Autodesk Fusion 360 part; units mm, degrees
(part 2 of 2)
sketch "Sketch5" plane through (0, 0, 12.2) normal (0, 0, 1) x (-1, 0, 0)
  circle A0 centre (8.13, -15.47) radius 0.762
  circle A1 centre (10.67, -18.01) radius 0.762
  circle A2 centre (8.13, -20.55) radius 0.762
  circle A3 centre (10.67, -23.09) radius 0.762
  circle A4 centre (8.13, -28.17) radius 0.762
  circle A5 centre (10.67, -25.63) radius 0.762
  circle A6 centre (10.67, -30.71) radius 0.762
  circle A7 centre (8.13, -33.25) radius 0.762
  circle A8 centre (10.67, -35.79) radius 0.762
  circle A9 centre (8.13, -38.33) radius 0.762
  circle A10 centre (13.21, -38.33) radius 0.762
  circle A11 centre (13.21, -33.25) radius 0.762
  circle A12 centre (13.21, -28.17) radius 0.762
  circle A13 centre (13.21, -23.09) radius 0.762
  circle A14 centre (13.21, -18.01) radius 0.762
  circle A15 centre (13.21, -12.93) radius 0.762
  circle A16 centre (8.13, -12.93) radius 0.762
  circle A17 centre (10.67, -10.39) radius 0.762
  circle A18 centre (13.21, -7.85) radius 0.762
  circle A19 centre (8.13, -7.85) radius 0.762
  circle A20 centre (5.59, -10.39) radius 0.762
  circle A21 centre (5.59, -15.47) radius 0.762
  circle A22 centre (5.59, -20.55) radius 0.762
  circle A23 centre (5.59, -25.63) radius 0.762
  circle A24 centre (5.59, -30.71) radius 0.762
  circle A25 centre (5.59, -35.79) radius 0.762
  circle A26 centre (3.05, -38.33) radius 0.762
  circle A27 centre (3.05, -33.25) radius 0.762
  circle A28 centre (3.05, -28.17) radius 0.762
  circle A29 centre (3.05, -23.09) radius 0.762
  circle A30 centre (3.05, -18.01) radius 0.762
  circle A31 centre (3.05, -12.93) radius 0.762
  circle A32 centre (3.05, -7.85) radius 0.762
  circle A33 centre (3.05, -5.31) radius 0.762
  circle A34 centre (5.59, -2.77) radius 0.762
  circle A35 centre (8.13, -5.31) radius 0.762
  circle A36 centre (13.21, -5.31) radius 0.762
  circle A37 centre (13.21, -2.77) radius 0.762
  circle A38 centre (13.21, 4.85) radius 0.762
  circle A39 centre (13.21, 7.39) radius 0.762
  circle A40 centre (10.67, 7.39) radius 0.762
  circle A41 centre (10.67, -0.23) radius 0.762
  circle A42 centre (8.13, 2.31) radius 0.762
  circle A43 centre (8.13, 7.39) radius 0.762
  circle A44 centre (5.59, 4.85) radius 0.762
  circle A45 centre (5.59, -0.23) radius 0.762
  circle A46 centre (3.05, -0.23) radius 0.762
  circle A47 centre (3.05, 7.39) radius 0.762
  circle A48 centre (5.59, 9.93) radius 0.762
  circle A49 centre (10.67, 9.93) radius 0.762
  circle A50 centre (13.21, 12.47) radius 0.762
  circle A51 centre (8.13, 12.47) radius 0.762
  circle A52 centre (8.13, 15.01) radius 0.762
  circle A53 centre (13.21, 15.01) radius 0.762
  circle A54 centre (13.21, 17.55) radius 0.762
  circle A55 centre (5.59, 20.09) radius 0.762
  circle A56 centre (8.13, 20.09) radius 0.762
  circle A57 centre (8.13, 22.63) radius 0.762
  circle A58 centre (3.05, 22.63) radius 0.762
  circle A59 centre (3.05, 17.55) radius 0.762
  circle A60 centre (3.05, 12.47) radius 0.762
  circle A61 centre (8.13, 17.55) radius 0.762
  circle A62 centre (13.21, 22.63) radius 0.762
  circle A63 centre (5.59, 27.71) radius 0.762
  circle A64 centre (3.05, 32.79) radius 0.762
  circle A65 centre (3.05, 27.71) radius 0.762
  circle A66 centre (5.59, 25.17) radius 0.762
  circle A67 centre (10.67, 25.17) radius 0.762
  circle A68 centre (8.13, 32.79) radius 0.762
  circle A69 centre (13.21, 32.79) radius 0.762
  circle A70 centre (13.21, 27.71) radius 0.762
  circle A71 centre (10.67, 27.71) radius 0.762
  circle A72 centre (5.59, 32.79) radius 0.762
  circle A73 centre (5.59, 35.33) radius 0.762
  circle A74 centre (10.67, 35.33) radius 0.762
  circle A75 centre (19.96, 23.9) radius 0.762
  circle A76 centre (19.96, 28.98) radius 0.762
  circle A77 centre (19.96, 34.06) radius 0.762
  circle A78 centre (22.5, 31.52) radius 0.762
  circle A79 centre (22.5, 26.44) radius 0.762
  circle A80 centre (22.5, 8.66) radius 0.762
  circle A81 centre (22.5, 13.74) radius 0.762
  circle A82 centre (22.5, 18.82) radius 0.762
  circle A83 centre (19.96, 16.28) radius 0.762
  circle A84 centre (19.96, 11.2) radius 0.762
  circle A85 centre (22.5, -6.58) radius 0.762
  circle A86 centre (22.5, -1.5) radius 0.762
  circle A87 centre (22.5, 3.58) radius 0.762
  circle A88 centre (19.96, 1.04) radius 0.762
  circle A89 centre (19.96, -4.04) radius 0.762
  circle A90 centre (22.5, -11.66) radius 0.762
  circle A91 centre (19.96, -14.2) radius 0.762
  circle A92 centre (22.5, -16.74) radius 0.762
  circle A93 centre (19.96, -19.28) radius 0.762
  circle A94 centre (22.5, -21.82) radius 0.762
  circle A95 centre (22.5, -34.52) radius 0.762
  circle A96 centre (22.5, -29.44) radius 0.762
  circle A97 centre (19.96, -26.9) radius 0.762
  circle A98 centre (19.96, -31.98) radius 0.762
  circle A99 centre (19.96, -37.06) radius 0.762
  circle A100 centre (22.5, -37.06) radius 0.762
  circle A101 centre (19.96, -34.52) radius 0.762
  circle A102 centre (19.96, -29.44) radius 0.762
  circle A103 centre (22.5, -26.9) radius 0.762
  circle A104 centre (22.5, -31.98) radius 0.762
  circle A105 centre (19.96, -21.82) radius 0.762
  circle A106 centre (22.5, -19.28) radius 0.762
  circle A107 centre (19.96, -16.74) radius 0.762
  circle A108 centre (22.5, -14.2) radius 0.762
  circle A109 centre (19.96, -11.66) radius 0.762
  circle A110 centre (19.96, -6.58) radius 0.762
  circle A111 centre (19.96, -1.5) radius 0.762
  circle A112 centre (19.96, 3.58) radius 0.762
  circle A113 centre (22.5, 1.04) radius 0.762
  circle A114 centre (22.5, -4.04) radius 0.762
  circle A115 centre (19.96, 8.66) radius 0.762
  circle A116 centre (19.96, 13.74) radius 0.762
  circle A117 centre (19.96, 18.82) radius 0.762
  circle A118 centre (22.5, 16.28) radius 0.762
  circle A119 centre (22.5, 11.2) radius 0.762
  circle A120 centre (22.5, 23.9) radius 0.762
  circle A121 centre (22.5, 28.98) radius 0.762
  circle A122 centre (22.5, 34.06) radius 0.762
  circle A123 centre (19.96, 31.52) radius 0.762
  circle A124 centre (19.96, 26.44) radius 0.762
  circle A125 centre (13.21, 35.33) radius 0.762
  circle A126 centre (8.13, 35.33) radius 0.762
  circle A127 centre (3.05, 35.33) radius 0.762
  circle A128 centre (8.13, 30.25) radius 0.762
  circle A129 centre (13.21, 25.17) radius 0.762
  circle A130 centre (13.21, 30.25) radius 0.762
  circle A131 centre (10.67, 32.79) radius 0.762
  circle A132 centre (10.67, 30.25) radius 0.762
  circle A133 centre (8.13, 25.17) radius 0.762
  circle A134 centre (3.05, 25.17) radius 0.762
  circle A135 centre (3.05, 30.25) radius 0.762
  circle A136 centre (5.59, 30.25) radius 0.762
  circle A137 centre (8.13, 27.71) radius 0.762
  circle A138 centre (10.67, 20.09) radius 0.762
  circle A139 centre (5.59, 15.01) radius 0.762
  circle A140 centre (3.05, 15.01) radius 0.762
  circle A141 centre (3.05, 20.09) radius 0.762
  circle A142 centre (5.59, 22.63) radius 0.762
  circle A143 centre (10.67, 22.63) radius 0.762
  circle A144 centre (5.59, 17.55) radius 0.762
  circle A145 centre (13.21, 20.09) radius 0.762
  circle A146 centre (10.67, 17.55) radius 0.762
  circle A147 centre (10.67, 15.01) radius 0.762
  circle A148 centre (5.59, 12.47) radius 0.762
  circle A149 centre (10.67, 12.47) radius 0.762
  circle A150 centre (13.21, 9.93) radius 0.762
  circle A151 centre (8.13, 9.93) radius 0.762
  circle A152 centre (3.05, 9.93) radius 0.762
  circle A153 centre (3.05, 4.85) radius 0.762
  circle A154 centre (3.05, 2.31) radius 0.762
  circle A155 centre (5.59, 2.31) radius 0.762
  circle A156 centre (5.59, 7.39) radius 0.762
  circle A157 centre (8.13, 4.85) radius 0.762
  circle A158 centre (8.13, -0.23) radius 0.762
  circle A159 centre (10.67, 2.31) radius 0.762
  circle A160 centre (10.67, 4.85) radius 0.762
  circle A161 centre (13.21, 2.31) radius 0.762
  circle A162 centre (13.21, -0.23) radius 0.762
  circle A163 centre (10.67, -5.31) radius 0.762
  circle A164 centre (10.67, -2.77) radius 0.762
  circle A165 centre (8.13, -2.77) radius 0.762
  circle A166 centre (5.59, -5.31) radius 0.762
  circle A167 centre (3.05, -2.77) radius 0.762
  circle A168 centre (3.05, -10.39) radius 0.762
  circle A169 centre (3.05, -15.47) radius 0.762
  circle A170 centre (3.05, -20.55) radius 0.762
  circle A171 centre (3.05, -25.63) radius 0.762
  circle A172 centre (3.05, -30.71) radius 0.762
  circle A173 centre (3.05, -35.79) radius 0.762
  circle A174 centre (5.59, -38.33) radius 0.762
  circle A175 centre (5.59, -33.25) radius 0.762
  circle A176 centre (5.59, -28.17) radius 0.762
  circle A177 centre (5.59, -23.09) radius 0.762
  circle A178 centre (5.59, -18.01) radius 0.762
  circle A179 centre (5.59, -12.93) radius 0.762
  circle A180 centre (5.59, -7.85) radius 0.762
  circle A181 centre (10.67, -7.85) radius 0.762
  circle A182 centre (13.21, -10.39) radius 0.762
  circle A183 centre (8.13, -10.39) radius 0.762
  circle A184 centre (10.67, -12.93) radius 0.762
  circle A185 centre (13.21, -15.47) radius 0.762
  circle A186 centre (13.21, -20.55) radius 0.762
  circle A187 centre (13.21, -25.63) radius 0.762
  circle A188 centre (13.21, -30.71) radius 0.762
  circle A189 centre (13.21, -35.79) radius 0.762
  circle A190 centre (10.67, -38.33) radius 0.762
  circle A191 centre (8.13, -35.79) radius 0.762
  circle A192 centre (10.67, -33.25) radius 0.762
  circle A193 centre (8.13, -30.71) radius 0.762
  circle A194 centre (10.67, -28.17) radius 0.762
  circle A195 centre (8.13, -25.63) radius 0.762
  circle A196 centre (8.13, -23.09) radius 0.762
  circle A197 centre (10.67, -20.55) radius 0.762
  circle A198 centre (8.13, -18.01) radius 0.762
  circle A199 centre (10.67, -15.47) radius 0.762
  line L0 (0.85, 38.65) -> (0.85, -41.65)
  line L1 (0.85, -41.65) -> (25.15, -41.65)
  line L2 (25.15, -41.65) -> (25.15, 38.65)
  line L3 (25.15, 38.65) -> (0.85, 38.65)
  circle A200 centre (-9.63, -2.77) radius 0.762
  circle A201 centre (-12.17, -5.31) radius 0.762
  circle A202 centre (-12.17, -0.23) radius 0.762
  circle A203 centre (-7.09, -0.23) radius 0.762
  circle A204 centre (-7.09, -5.31) radius 0.762
  circle A205 centre (-9.63, -7.85) radius 0.762
  circle A206 centre (-12.17, -10.39) radius 0.762
  circle A207 centre (-7.09, -10.39) radius 0.762
  circle A208 centre (-9.63, 2.31) radius 0.762
  circle A209 centre (-12.17, 4.85) radius 0.762
  circle A210 centre (-7.09, 4.85) radius 0.762
  circle A211 centre (-9.63, 7.39) radius 0.762
  circle A212 centre (-12.17, 9.93) radius 0.762
  circle A213 centre (-7.09, 9.93) radius 0.762
  circle A214 centre (-9.63, 12.47) radius 0.762
  circle A215 centre (-12.17, 15.01) radius 0.762
  circle A216 centre (-7.09, 15.01) radius 0.762
  circle A217 centre (-9.63, 17.55) radius 0.762
  circle A218 centre (-14.71, -10.39) radius 0.762
  circle A219 centre (-14.71, -5.31) radius 0.762
  circle A220 centre (-14.71, 2.31) radius 0.762
  circle A221 centre (-14.71, 4.85) radius 0.762
  circle A222 centre (-14.71, 9.93) radius 0.762
  circle A223 centre (-14.71, 15.01) radius 0.762
  circle A224 centre (-4.55, 17.55) radius 0.762
  circle A225 centre (-4.55, 12.47) radius 0.762
  circle A226 centre (-4.55, 7.39) radius 0.762
  circle A227 centre (-4.55, 2.31) radius 0.762
  circle A228 centre (-4.55, -2.77) radius 0.762
  circle A229 centre (-4.55, -7.85) radius 0.762
  circle A230 centre (-4.55, -12.93) radius 0.762
  circle A231 centre (-9.63, -12.93) radius 0.762
  circle A232 centre (-14.71, -12.93) radius 0.762
  circle A233 centre (-12.17, -15.47) radius 0.762
  circle A234 centre (-7.09, -15.47) radius 0.762
  circle A235 centre (-4.55, -18.01) radius 0.762
  circle A236 centre (-9.63, -18.01) radius 0.762
  circle A237 centre (-14.71, -18.01) radius 0.762
  circle A238 centre (-14.71, -23.09) radius 0.762
  circle A239 centre (-12.17, -20.55) radius 0.762
  circle A240 centre (-9.63, -23.09) radius 0.762
  circle A241 centre (-12.17, -25.63) radius 0.762
  circle A242 centre (-14.71, -28.17) radius 0.762
  circle A243 centre (-9.63, -28.17) radius 0.762
  circle A244 centre (-7.09, -25.63) radius 0.762
  circle A245 centre (-7.09, -20.55) radius 0.762
  circle A246 centre (-4.55, -23.09) radius 0.762
  circle A247 centre (-4.55, -28.17) radius 0.762
  circle A248 centre (-7.09, -30.71) radius 0.762
  circle A249 centre (-12.17, -30.71) radius 0.762
  circle A250 centre (-14.71, -33.25) radius 0.762
  circle A251 centre (-9.63, -33.25) radius 0.762
  circle A252 centre (-4.55, -33.25) radius 0.762
  circle A253 centre (-12.17, 20.09) radius 0.762
  circle A254 centre (-7.09, 20.09) radius 0.762
  circle A255 centre (-4.55, 22.63) radius 0.762
  circle A256 centre (-4.55, 27.71) radius 0.762
  circle A257 centre (-7.09, 25.17) radius 0.762
  circle A258 centre (-9.63, 22.63) radius 0.762
  circle A259 centre (-9.63, 27.71) radius 0.762
  circle A260 centre (-12.17, 25.17) radius 0.762
  circle A261 centre (-14.71, 22.63) radius 0.762
  circle A262 centre (-14.71, 27.71) radius 0.762
  circle A263 centre (-12.17, 30.25) radius 0.762
  circle A264 centre (-7.09, 30.25) radius 0.762
  circle A265 centre (-4.55, 32.79) radius 0.762
  circle A266 centre (-9.63, 32.79) radius 0.762
  circle A267 centre (-14.71, 32.79) radius 0.762
  circle A268 centre (-12.17, 35.33) radius 0.762
  circle A269 centre (-7.09, 35.33) radius 0.762
  circle A270 centre (-4.55, -35.79) radius 0.762
  circle A271 centre (-9.63, -35.79) radius 0.762
  circle A272 centre (-14.71, -35.79) radius 0.762
  circle A273 centre (-12.17, -38.33) radius 0.762
  circle A274 centre (-7.09, -38.33) radius 0.762
  circle A275 centre (-21.46, -37.06) radius 0.762
  circle A276 centre (-24, -34.52) radius 0.762
  circle A277 centre (-21.46, -31.98) radius 0.762
  circle A278 centre (-24, -29.44) radius 0.762
  circle A279 centre (-21.46, -26.9) radius 0.762
  circle A280 centre (-24, -21.82) radius 0.762
  circle A281 centre (-21.46, -19.28) radius 0.762
  circle A282 centre (-24, -16.74) radius 0.762
  circle A283 centre (-21.46, -14.2) radius 0.762
  circle A284 centre (-24, -11.66) radius 0.762
  circle A285 centre (-21.46, 26.44) radius 0.762
  circle A286 centre (-21.46, 31.52) radius 0.762
  circle A287 centre (-24, 34.06) radius 0.762
  circle A288 centre (-24, 28.98) radius 0.762
  circle A289 centre (-24, 23.9) radius 0.762
  circle A290 centre (-21.46, 18.82) radius 0.762
  circle A291 centre (-24, 16.28) radius 0.762
  circle A292 centre (-21.46, 13.74) radius 0.762
  circle A293 centre (-24, 11.2) radius 0.762
  circle A294 centre (-21.46, 8.66) radius 0.762
  circle A295 centre (-24, 3.58) radius 0.762
  circle A296 centre (-21.46, 1.04) radius 0.762
  circle A297 centre (-24, -1.5) radius 0.762
  circle A298 centre (-21.46, -4.04) radius 0.762
  circle A299 centre (-24, -6.58) radius 0.762
  circle A300 centre (-21.46, -6.58) radius 0.762
  circle A301 centre (-24, -4.04) radius 0.762
  circle A302 centre (-21.46, -1.5) radius 0.762
  circle A303 centre (-24, 1.04) radius 0.762
  circle A304 centre (-21.46, 3.58) radius 0.762
  circle A305 centre (-24, 8.66) radius 0.762
  circle A306 centre (-21.46, 11.2) radius 0.762
  circle A307 centre (-24, 13.74) radius 0.762
  circle A308 centre (-21.46, 16.28) radius 0.762
  circle A309 centre (-24, 18.82) radius 0.762
  circle A310 centre (-21.46, 23.9) radius 0.762
  circle A311 centre (-24, 26.44) radius 0.762
  circle A312 centre (-24, 31.52) radius 0.762
  circle A313 centre (-21.46, 34.06) radius 0.762
  circle A314 centre (-21.46, 28.98) radius 0.762
  circle A315 centre (-21.46, -11.66) radius 0.762
  circle A316 centre (-24, -14.2) radius 0.762
  circle A317 centre (-21.46, -16.74) radius 0.762
  circle A318 centre (-24, -19.28) radius 0.762
  circle A319 centre (-21.46, -21.82) radius 0.762
  circle A320 centre (-24, -26.9) radius 0.762
  circle A321 centre (-21.46, -29.44) radius 0.762
  circle A322 centre (-24, -31.98) radius 0.762
  circle A323 centre (-21.46, -34.52) radius 0.762
  circle A324 centre (-24, -37.06) radius 0.762
  circle A325 centre (-4.55, -38.33) radius 0.762
  circle A326 centre (-9.63, -38.33) radius 0.762
  circle A327 centre (-14.71, -38.33) radius 0.762
  circle A328 centre (-12.17, -35.79) radius 0.762
  circle A329 centre (-7.09, -35.79) radius 0.762
  circle A330 centre (-4.55, 35.33) radius 0.762
  circle A331 centre (-9.63, 35.33) radius 0.762
  circle A332 centre (-14.71, 35.33) radius 0.762
  circle A333 centre (-12.17, 32.79) radius 0.762
  circle A334 centre (-7.09, 32.79) radius 0.762
  circle A335 centre (-4.55, 30.25) radius 0.762
  circle A336 centre (-9.63, 30.25) radius 0.762
  circle A337 centre (-14.71, 30.25) radius 0.762
  circle A338 centre (-14.71, 25.17) radius 0.762
  circle A339 centre (-12.17, 22.63) radius 0.762
  circle A340 centre (-12.17, 27.71) radius 0.762
  circle A341 centre (-9.63, 25.17) radius 0.762
  circle A342 centre (-7.09, 22.63) radius 0.762
  circle A343 centre (-7.09, 27.71) radius 0.762
  circle A344 centre (-4.55, 25.17) radius 0.762
  circle A345 centre (-4.55, 20.09) radius 0.762
  circle A346 centre (-9.63, 20.09) radius 0.762
  circle A347 centre (-14.71, 20.09) radius 0.762
  circle A348 centre (-7.09, -33.25) radius 0.762
  circle A349 centre (-12.17, -33.25) radius 0.762
  circle A350 centre (-14.71, -30.71) radius 0.762
  circle A351 centre (-9.63, -30.71) radius 0.762
  circle A352 centre (-4.55, -30.71) radius 0.762
  circle A353 centre (-4.55, -25.63) radius 0.762
  circle A354 centre (-4.55, -20.55) radius 0.762
  circle A355 centre (-7.09, -23.09) radius 0.762
  circle A356 centre (-7.09, -28.17) radius 0.762
  circle A357 centre (-12.17, -28.17) radius 0.762
  circle A358 centre (-14.71, -25.63) radius 0.762
  circle A359 centre (-9.63, -25.63) radius 0.762
  circle A360 centre (-9.63, -20.55) radius 0.762
  circle A361 centre (-12.17, -23.09) radius 0.762
  circle A362 centre (-14.71, -20.55) radius 0.762
  circle A363 centre (-12.17, -18.01) radius 0.762
  circle A364 centre (-7.09, -18.01) radius 0.762
  circle A365 centre (-4.55, -15.47) radius 0.762
  circle A366 centre (-9.63, -15.47) radius 0.762
  circle A367 centre (-14.71, -15.47) radius 0.762
  circle A368 centre (-12.17, -12.93) radius 0.762
  circle A369 centre (-7.09, -12.93) radius 0.762
  circle A370 centre (-4.55, -10.39) radius 0.762
  circle A371 centre (-4.55, -5.31) radius 0.762
  circle A372 centre (-4.55, -0.23) radius 0.762
  circle A373 centre (-4.55, 4.85) radius 0.762
  circle A374 centre (-4.55, 9.93) radius 0.762
  circle A375 centre (-4.55, 15.01) radius 0.762
  circle A376 centre (-14.71, 17.55) radius 0.762
  circle A377 centre (-14.71, 12.47) radius 0.762
  circle A378 centre (-14.71, 7.39) radius 0.762
  circle A379 centre (-14.71, -0.23) radius 0.762
  circle A380 centre (-14.71, -2.77) radius 0.762
  circle A381 centre (-14.71, -7.85) radius 0.762
  circle A382 centre (-12.17, 17.55) radius 0.762
  circle A383 centre (-7.09, 17.55) radius 0.762
  circle A384 centre (-9.63, 15.01) radius 0.762
  circle A385 centre (-12.17, 12.47) radius 0.762
  circle A386 centre (-7.09, 12.47) radius 0.762
  circle A387 centre (-9.63, 9.93) radius 0.762
  circle A388 centre (-12.17, 7.39) radius 0.762
  circle A389 centre (-7.09, 7.39) radius 0.762
  circle A390 centre (-9.63, 4.85) radius 0.762
  circle A391 centre (-12.17, 2.31) radius 0.762
  circle A392 centre (-7.09, 2.31) radius 0.762
  circle A393 centre (-9.63, -10.39) radius 0.762
  circle A394 centre (-7.09, -7.85) radius 0.762
  circle A395 centre (-12.17, -7.85) radius 0.762
  circle A396 centre (-7.09, -2.77) radius 0.762
  circle A397 centre (-9.63, -0.23) radius 0.762
  circle A398 centre (-12.17, -2.77) radius 0.762
  circle A399 centre (-9.63, -5.31) radius 0.762
  line L4 (-2.35, 38.65) -> (-26.65, 38.65)
  line L5 (-26.65, 38.65) -> (-26.65, -41.65)
  line L6 (-26.65, -41.65) -> (-2.35, -41.65)
  line L7 (-2.35, -41.65) -> (-2.35, 38.65)
  point P0 (3.8, -1.27)
  point P1 (6.34, -1.27)
  point P2 (8.88, -1.27)
  point P3 (11.42, -1.27)
  point P4 (13.96, -1.27)
  point P5 (3.8, -3.81)
  point P6 (6.34, -3.81)
  point P7 (8.88, -3.81)
  point P8 (11.42, -3.81)
  point P9 (13.96, -3.81)
  point P10 (3.8, -6.35)
  point P11 (6.34, -6.35)
  point P12 (8.88, -6.35)
  point P13 (11.42, -6.35)
  point P14 (13.96, -6.35)
  point P15 (3.8, -8.89)
  point P16 (6.34, -8.89)
  point P17 (8.88, -8.89)
  point P18 (11.42, -8.89)
  point P19 (13.96, -8.89)
  point P20 (3.8, -11.43)
  point P21 (6.34, -11.43)
  point P22 (8.88, -11.43)
  point P23 (11.42, -11.43)
  point P24 (13.96, -11.43)
  point P25 (3.8, -13.97)
  point P26 (6.34, -13.97)
  point P27 (8.88, -13.97)
  point P28 (11.42, -13.97)
  point P29 (13.96, -13.97)
  point P30 (3.8, -16.51)
  point P31 (6.34, -16.51)
  point P32 (8.88, -16.51)
  point P33 (11.42, -16.51)
  point P34 (13.96, -16.51)
  point P35 (3.8, -19.05)
  point P36 (6.34, -19.05)
  point P37 (8.88, -19.05)
  point P38 (11.42, -19.05)
  point P39 (13.96, -19.05)
  point P40 (3.8, -21.59)
  point P41 (6.34, -21.59)
  point P42 (8.88, -21.59)
  point P43 (11.42, -21.59)
  point P44 (13.96, -21.59)
  point P45 (3.8, -24.13)
  point P46 (6.34, -24.13)
  point P47 (8.88, -24.13)
  point P48 (11.42, -24.13)
  point P49 (13.96, -24.13)
  point P50 (3.8, -26.67)
  point P51 (6.34, -26.67)
  point P52 (8.88, -26.67)
  point P53 (11.42, -26.67)
  point P54 (13.96, -26.67)
  point P55 (3.8, -29.21)
  point P56 (6.34, -29.21)
  point P57 (8.88, -29.21)
  point P58 (11.42, -29.21)
  point P59 (13.96, -29.21)
  point P60 (3.8, -31.75)
  point P61 (6.34, -31.75)
  point P62 (8.88, -31.75)
  point P63 (11.42, -31.75)
  point P64 (13.96, -31.75)
  point P65 (3.8, -34.29)
  point P66 (6.34, -34.29)
  point P67 (8.88, -34.29)
  point P68 (11.42, -34.29)
  point P69 (13.96, -34.29)
  point P70 (3.8, -36.83)
  point P71 (6.34, -36.83)
  point P72 (8.88, -36.83)
  point P73 (11.42, -36.83)
  point P74 (13.96, -36.83)
  dimension "d31" = 3.8
  dimension "d32" = 1.27
  dimension "d35" = 10.16
  dimension "d36" = -35.56
  measures "d31" horizontal distance of origin P0
  measures "d32" vertical distance of origin P0
sketch "Sketch6" plane through (0, 0, 12.2) normal (0, 0, 1) x (-1, 0, 0)
  line L0 (0, 0) -> (26.398, 0) construction
  circle A0 centre (8.13, -15.47) radius 0.762
  circle A1 centre (10.67, -18.01) radius 0.762
  circle A2 centre (8.13, -20.55) radius 0.762
  circle A3 centre (10.67, -23.09) radius 0.762
  circle A4 centre (8.13, -28.17) radius 0.762
  circle A5 centre (10.67, -25.63) radius 0.762
  circle A6 centre (10.67, -30.71) radius 0.762
  circle A7 centre (8.13, -33.25) radius 0.762
  circle A8 centre (10.67, -35.79) radius 0.762
  circle A9 centre (8.13, -38.33) radius 0.762
  circle A10 centre (13.21, -38.33) radius 0.762
  circle A11 centre (13.21, -33.25) radius 0.762
  circle A12 centre (13.21, -28.17) radius 0.762
  circle A13 centre (13.21, -23.09) radius 0.762
  circle A14 centre (13.21, -18.01) radius 0.762
  circle A15 centre (13.21, -12.93) radius 0.762
  circle A16 centre (8.13, -12.93) radius 0.762
  circle A17 centre (10.67, -10.39) radius 0.762
  circle A18 centre (13.21, -7.85) radius 0.762
  circle A19 centre (8.13, -7.85) radius 0.762
  circle A20 centre (5.59, -10.39) radius 0.762
  circle A21 centre (5.59, -15.47) radius 0.762
  circle A22 centre (5.59, -20.55) radius 0.762
  circle A23 centre (5.59, -25.63) radius 0.762
  circle A24 centre (5.59, -30.71) radius 0.762
  circle A25 centre (5.59, -35.79) radius 0.762
  circle A26 centre (3.05, -38.33) radius 0.762
  circle A27 centre (3.05, -33.25) radius 0.762
  circle A28 centre (3.05, -28.17) radius 0.762
  circle A29 centre (3.05, -23.09) radius 0.762
  circle A30 centre (3.05, -18.01) radius 0.762
  circle A31 centre (3.05, -12.93) radius 0.762
  circle A32 centre (3.05, -7.85) radius 0.762
  circle A33 centre (3.05, -5.31) radius 0.762
  circle A34 centre (5.59, -2.77) radius 0.762
  circle A35 centre (8.13, -5.31) radius 0.762
  circle A36 centre (13.21, -5.31) radius 0.762
  circle A37 centre (13.21, -2.77) radius 0.762
  circle A38 centre (13.21, 4.85) radius 0.762
  circle A39 centre (13.21, 7.39) radius 0.762
  circle A40 centre (10.67, 7.39) radius 0.762
  circle A41 centre (10.67, -0.23) radius 0.762
  circle A42 centre (8.13, 2.31) radius 0.762
  circle A43 centre (8.13, 7.39) radius 0.762
  circle A44 centre (5.59, 4.85) radius 0.762
  circle A45 centre (5.59, -0.23) radius 0.762
  circle A46 centre (3.05, -0.23) radius 0.762
  circle A47 centre (3.05, 7.39) radius 0.762
  circle A48 centre (5.59, 9.93) radius 0.762
  circle A49 centre (10.67, 9.93) radius 0.762
  circle A50 centre (13.21, 12.47) radius 0.762
  circle A51 centre (8.13, 12.47) radius 0.762
  circle A52 centre (8.13, 15.01) radius 0.762
  circle A53 centre (13.21, 15.01) radius 0.762
  circle A54 centre (13.21, 17.55) radius 0.762
  circle A55 centre (5.59, 20.09) radius 0.762
  circle A56 centre (8.13, 20.09) radius 0.762
  circle A57 centre (8.13, 22.63) radius 0.762
  circle A58 centre (3.05, 22.63) radius 0.762
  circle A59 centre (3.05, 17.55) radius 0.762
  circle A60 centre (3.05, 12.47) radius 0.762
  circle A61 centre (8.13, 17.55) radius 0.762
  circle A62 centre (13.21, 22.63) radius 0.762
  circle A63 centre (5.59, 27.71) radius 0.762
  circle A64 centre (3.05, 32.79) radius 0.762
  circle A65 centre (3.05, 27.71) radius 0.762
  circle A66 centre (5.59, 25.17) radius 0.762
  circle A67 centre (10.67, 25.17) radius 0.762
  circle A68 centre (8.13, 32.79) radius 0.762
  circle A69 centre (13.21, 32.79) radius 0.762
  circle A70 centre (13.21, 27.71) radius 0.762
  circle A71 centre (10.67, 27.71) radius 0.762
  circle A72 centre (5.59, 32.79) radius 0.762
  circle A73 centre (5.59, 35.33) radius 0.762
  circle A74 centre (10.67, 35.33) radius 0.762
  circle A75 centre (19.96, 23.9) radius 0.762
  circle A76 centre (19.96, 28.98) radius 0.762
  circle A77 centre (19.96, 34.06) radius 0.762
  circle A78 centre (22.5, 31.52) radius 0.762
  circle A79 centre (22.5, 26.44) radius 0.762
  circle A80 centre (22.5, 8.66) radius 0.762
  circle A81 centre (22.5, 13.74) radius 0.762
  circle A82 centre (22.5, 18.82) radius 0.762
  circle A83 centre (19.96, 16.28) radius 0.762
  circle A84 centre (19.96, 11.2) radius 0.762
  circle A85 centre (22.5, -6.58) radius 0.762
  circle A86 centre (22.5, -1.5) radius 0.762
  circle A87 centre (22.5, 3.58) radius 0.762
  circle A88 centre (19.96, 1.04) radius 0.762
  circle A89 centre (19.96, -4.04) radius 0.762
  circle A90 centre (22.5, -11.66) radius 0.762
  circle A91 centre (19.96, -14.2) radius 0.762
  circle A92 centre (22.5, -16.74) radius 0.762
  circle A93 centre (19.96, -19.28) radius 0.762
  circle A94 centre (22.5, -21.82) radius 0.762
  circle A95 centre (22.5, -34.52) radius 0.762
  circle A96 centre (22.5, -29.44) radius 0.762
  circle A97 centre (19.96, -26.9) radius 0.762
  circle A98 centre (19.96, -31.98) radius 0.762
  circle A99 centre (19.96, -37.06) radius 0.762
  circle A100 centre (22.5, -37.06) radius 0.762
  circle A101 centre (19.96, -34.52) radius 0.762
  circle A102 centre (19.96, -29.44) radius 0.762
  circle A103 centre (22.5, -26.9) radius 0.762
  circle A104 centre (22.5, -31.98) radius 0.762
  circle A105 centre (19.96, -21.82) radius 0.762
  circle A106 centre (22.5, -19.28) radius 0.762
  circle A107 centre (19.96, -16.74) radius 0.762
  circle A108 centre (22.5, -14.2) radius 0.762
  circle A109 centre (19.96, -11.66) radius 0.762
  circle A110 centre (19.96, -6.58) radius 0.762
  circle A111 centre (19.96, -1.5) radius 0.762
  circle A112 centre (19.96, 3.58) radius 0.762
  circle A113 centre (22.5, 1.04) radius 0.762
  circle A114 centre (22.5, -4.04) radius 0.762
  circle A115 centre (19.96, 8.66) radius 0.762
  circle A116 centre (19.96, 13.74) radius 0.762
  circle A117 centre (19.96, 18.82) radius 0.762
  circle A118 centre (22.5, 16.28) radius 0.762
  circle A119 centre (22.5, 11.2) radius 0.762
  circle A120 centre (22.5, 23.9) radius 0.762
  circle A121 centre (22.5, 28.98) radius 0.762
  circle A122 centre (22.5, 34.06) radius 0.762
  circle A123 centre (19.96, 31.52) radius 0.762
  circle A124 centre (19.96, 26.44) radius 0.762
  circle A125 centre (13.21, 35.33) radius 0.762
  circle A126 centre (8.13, 35.33) radius 0.762
  circle A127 centre (3.05, 35.33) radius 0.762
  circle A128 centre (8.13, 30.25) radius 0.762
  circle A129 centre (13.21, 25.17) radius 0.762
  circle A130 centre (13.21, 30.25) radius 0.762
  circle A131 centre (10.67, 32.79) radius 0.762
  circle A132 centre (10.67, 30.25) radius 0.762
  circle A133 centre (8.13, 25.17) radius 0.762
  circle A134 centre (3.05, 25.17) radius 0.762
  circle A135 centre (3.05, 30.25) radius 0.762
  circle A136 centre (5.59, 30.25) radius 0.762
  circle A137 centre (8.13, 27.71) radius 0.762
  circle A138 centre (10.67, 20.09) radius 0.762
  circle A139 centre (5.59, 15.01) radius 0.762
  circle A140 centre (3.05, 15.01) radius 0.762
  circle A141 centre (3.05, 20.09) radius 0.762
  circle A142 centre (5.59, 22.63) radius 0.762
  circle A143 centre (10.67, 22.63) radius 0.762
  circle A144 centre (5.59, 17.55) radius 0.762
  circle A145 centre (13.21, 20.09) radius 0.762
  circle A146 centre (10.67, 17.55) radius 0.762
  circle A147 centre (10.67, 15.01) radius 0.762
  circle A148 centre (5.59, 12.47) radius 0.762
  circle A149 centre (10.67, 12.47) radius 0.762
  circle A150 centre (13.21, 9.93) radius 0.762
  circle A151 centre (8.13, 9.93) radius 0.762
  circle A152 centre (3.05, 9.93) radius 0.762
  circle A153 centre (3.05, 4.85) radius 0.762
  circle A154 centre (3.05, 2.31) radius 0.762
  circle A155 centre (5.59, 2.31) radius 0.762
  circle A156 centre (5.59, 7.39) radius 0.762
  circle A157 centre (8.13, 4.85) radius 0.762
  circle A158 centre (8.13, -0.23) radius 0.762
  circle A159 centre (10.67, 2.31) radius 0.762
  circle A160 centre (10.67, 4.85) radius 0.762
  circle A161 centre (13.21, 2.31) radius 0.762
  circle A162 centre (13.21, -0.23) radius 0.762
  circle A163 centre (10.67, -5.31) radius 0.762
  circle A164 centre (10.67, -2.77) radius 0.762
  circle A165 centre (8.13, -2.77) radius 0.762
  circle A166 centre (5.59, -5.31) radius 0.762
  circle A167 centre (3.05, -2.77) radius 0.762
  circle A168 centre (3.05, -10.39) radius 0.762
  circle A169 centre (3.05, -15.47) radius 0.762
  circle A170 centre (3.05, -20.55) radius 0.762
  circle A171 centre (3.05, -25.63) radius 0.762
  circle A172 centre (3.05, -30.71) radius 0.762
  circle A173 centre (3.05, -35.79) radius 0.762
  circle A174 centre (5.59, -38.33) radius 0.762
  circle A175 centre (5.59, -33.25) radius 0.762
  circle A176 centre (5.59, -28.17) radius 0.762
  circle A177 centre (5.59, -23.09) radius 0.762
  circle A178 centre (5.59, -18.01) radius 0.762
  circle A179 centre (5.59, -12.93) radius 0.762
  circle A180 centre (5.59, -7.85) radius 0.762
  circle A181 centre (10.67, -7.85) radius 0.762
  circle A182 centre (13.21, -10.39) radius 0.762
  circle A183 centre (8.13, -10.39) radius 0.762
  circle A184 centre (10.67, -12.93) radius 0.762
  circle A185 centre (13.21, -15.47) radius 0.762
  circle A186 centre (13.21, -20.55) radius 0.762
  circle A187 centre (13.21, -25.63) radius 0.762
  circle A188 centre (13.21, -30.71) radius 0.762
  circle A189 centre (13.21, -35.79) radius 0.762
  circle A190 centre (10.67, -38.33) radius 0.762
  circle A191 centre (8.13, -35.79) radius 0.762
  circle A192 centre (10.67, -33.25) radius 0.762
  circle A193 centre (8.13, -30.71) radius 0.762
  circle A194 centre (10.67, -28.17) radius 0.762
  circle A195 centre (8.13, -25.63) radius 0.762
  circle A196 centre (8.13, -23.09) radius 0.762
  circle A197 centre (10.67, -20.55) radius 0.762
  circle A198 centre (8.13, -18.01) radius 0.762
  circle A199 centre (10.67, -15.47) radius 0.762
  line L1 (0.85, 38.65) -> (0.85, -41.65)
  line L2 (0.85, -41.65) -> (25.15, -41.65)
  line L3 (25.15, -41.65) -> (25.15, 38.65)
  line L4 (25.15, 38.65) -> (0.85, 38.65)
  circle A200 centre (-9.63, -2.77) radius 0.762
  circle A201 centre (-12.17, -5.31) radius 0.762
  circle A202 centre (-12.17, -0.23) radius 0.762
  circle A203 centre (-7.09, -0.23) radius 0.762
  circle A204 centre (-7.09, -5.31) radius 0.762
  circle A205 centre (-9.63, -7.85) radius 0.762
  circle A206 centre (-12.17, -10.39) radius 0.762
  circle A207 centre (-7.09, -10.39) radius 0.762
  circle A208 centre (-9.63, 2.31) radius 0.762
  circle A209 centre (-12.17, 4.85) radius 0.762
  circle A210 centre (-7.09, 4.85) radius 0.762
  circle A211 centre (-9.63, 7.39) radius 0.762
  circle A212 centre (-12.17, 9.93) radius 0.762
  circle A213 centre (-7.09, 9.93) radius 0.762
  circle A214 centre (-9.63, 12.47) radius 0.762
  circle A215 centre (-12.17, 15.01) radius 0.762
  circle A216 centre (-7.09, 15.01) radius 0.762
  circle A217 centre (-9.63, 17.55) radius 0.762
  circle A218 centre (-14.71, -10.39) radius 0.762
  circle A219 centre (-14.71, -5.31) radius 0.762
  circle A220 centre (-14.71, 2.31) radius 0.762
  circle A221 centre (-14.71, 4.85) radius 0.762
  circle A222 centre (-14.71, 9.93) radius 0.762
  circle A223 centre (-14.71, 15.01) radius 0.762
  circle A224 centre (-4.55, 17.55) radius 0.762
  circle A225 centre (-4.55, 12.47) radius 0.762
  circle A226 centre (-4.55, 7.39) radius 0.762
  circle A227 centre (-4.55, 2.31) radius 0.762
  circle A228 centre (-4.55, -2.77) radius 0.762
  circle A229 centre (-4.55, -7.85) radius 0.762
  circle A230 centre (-4.55, -12.93) radius 0.762
  circle A231 centre (-9.63, -12.93) radius 0.762
  circle A232 centre (-14.71, -12.93) radius 0.762
  circle A233 centre (-12.17, -15.47) radius 0.762
  circle A234 centre (-7.09, -15.47) radius 0.762
  circle A235 centre (-4.55, -18.01) radius 0.762
  circle A236 centre (-9.63, -18.01) radius 0.762
  circle A237 centre (-14.71, -18.01) radius 0.762
  circle A238 centre (-14.71, -23.09) radius 0.762
  circle A239 centre (-12.17, -20.55) radius 0.762
  circle A240 centre (-9.63, -23.09) radius 0.762
  circle A241 centre (-12.17, -25.63) radius 0.762
  circle A242 centre (-14.71, -28.17) radius 0.762
  circle A243 centre (-9.63, -28.17) radius 0.762
  circle A244 centre (-7.09, -25.63) radius 0.762
  circle A245 centre (-7.09, -20.55) radius 0.762
  circle A246 centre (-4.55, -23.09) radius 0.762
  circle A247 centre (-4.55, -28.17) radius 0.762
  circle A248 centre (-7.09, -30.71) radius 0.762
  circle A249 centre (-12.17, -30.71) radius 0.762
  circle A250 centre (-14.71, -33.25) radius 0.762
  circle A251 centre (-9.63, -33.25) radius 0.762
  circle A252 centre (-4.55, -33.25) radius 0.762
  circle A253 centre (-12.17, 20.09) radius 0.762
  circle A254 centre (-7.09, 20.09) radius 0.762
  circle A255 centre (-4.55, 22.63) radius 0.762
  circle A256 centre (-4.55, 27.71) radius 0.762
  circle A257 centre (-7.09, 25.17) radius 0.762
  circle A258 centre (-9.63, 22.63) radius 0.762
  circle A259 centre (-9.63, 27.71) radius 0.762
  circle A260 centre (-12.17, 25.17) radius 0.762
  circle A261 centre (-14.71, 22.63) radius 0.762
  circle A262 centre (-14.71, 27.71) radius 0.762
  circle A263 centre (-12.17, 30.25) radius 0.762
  circle A264 centre (-7.09, 30.25) radius 0.762
  circle A265 centre (-4.55, 32.79) radius 0.762
  circle A266 centre (-9.63, 32.79) radius 0.762
  circle A267 centre (-14.71, 32.79) radius 0.762
  circle A268 centre (-12.17, 35.33) radius 0.762
  circle A269 centre (-7.09, 35.33) radius 0.762
  circle A270 centre (-4.55, -35.79) radius 0.762
  circle A271 centre (-9.63, -35.79) radius 0.762
  circle A272 centre (-14.71, -35.79) radius 0.762
  circle A273 centre (-12.17, -38.33) radius 0.762
  circle A274 centre (-7.09, -38.33) radius 0.762
  circle A275 centre (-21.46, -37.06) radius 0.762
  circle A276 centre (-24, -34.52) radius 0.762
  circle A277 centre (-21.46, -31.98) radius 0.762
  circle A278 centre (-24, -29.44) radius 0.762
  circle A279 centre (-21.46, -26.9) radius 0.762
  circle A280 centre (-24, -21.82) radius 0.762
  circle A281 centre (-21.46, -19.28) radius 0.762
  circle A282 centre (-24, -16.74) radius 0.762
  circle A283 centre (-21.46, -14.2) radius 0.762
  circle A284 centre (-24, -11.66) radius 0.762
  circle A285 centre (-21.46, 26.44) radius 0.762
  circle A286 centre (-21.46, 31.52) radius 0.762
  circle A287 centre (-24, 34.06) radius 0.762
  circle A288 centre (-24, 28.98) radius 0.762
  circle A289 centre (-24, 23.9) radius 0.762
  circle A290 centre (-21.46, 18.82) radius 0.762
  circle A291 centre (-24, 16.28) radius 0.762
  circle A292 centre (-21.46, 13.74) radius 0.762
  circle A293 centre (-24, 11.2) radius 0.762
  circle A294 centre (-21.46, 8.66) radius 0.762
  circle A295 centre (-24, 3.58) radius 0.762
  circle A296 centre (-21.46, 1.04) radius 0.762
  circle A297 centre (-24, -1.5) radius 0.762
  circle A298 centre (-21.46, -4.04) radius 0.762
  circle A299 centre (-24, -6.58) radius 0.762
  circle A300 centre (-21.46, -6.58) radius 0.762
  circle A301 centre (-24, -4.04) radius 0.762
  circle A302 centre (-21.46, -1.5) radius 0.762
  circle A303 centre (-24, 1.04) radius 0.762
  circle A304 centre (-21.46, 3.58) radius 0.762
  circle A305 centre (-24, 8.66) radius 0.762
  circle A306 centre (-21.46, 11.2) radius 0.762
  circle A307 centre (-24, 13.74) radius 0.762
  circle A308 centre (-21.46, 16.28) radius 0.762
  circle A309 centre (-24, 18.82) radius 0.762
  circle A310 centre (-21.46, 23.9) radius 0.762
  circle A311 centre (-24, 26.44) radius 0.762
  circle A312 centre (-24, 31.52) radius 0.762
  circle A313 centre (-21.46, 34.06) radius 0.762
  circle A314 centre (-21.46, 28.98) radius 0.762
  circle A315 centre (-21.46, -11.66) radius 0.762
  circle A316 centre (-24, -14.2) radius 0.762
  circle A317 centre (-21.46, -16.74) radius 0.762
  circle A318 centre (-24, -19.28) radius 0.762
  circle A319 centre (-21.46, -21.82) radius 0.762
  circle A320 centre (-24, -26.9) radius 0.762
  circle A321 centre (-21.46, -29.44) radius 0.762
  circle A322 centre (-24, -31.98) radius 0.762
  circle A323 centre (-21.46, -34.52) radius 0.762
  circle A324 centre (-24, -37.06) radius 0.762
  circle A325 centre (-4.55, -38.33) radius 0.762
  circle A326 centre (-9.63, -38.33) radius 0.762
  circle A327 centre (-14.71, -38.33) radius 0.762
  circle A328 centre (-12.17, -35.79) radius 0.762
  circle A329 centre (-7.09, -35.79) radius 0.762
  circle A330 centre (-4.55, 35.33) radius 0.762
  circle A331 centre (-9.63, 35.33) radius 0.762
  circle A332 centre (-14.71, 35.33) radius 0.762
  circle A333 centre (-12.17, 32.79) radius 0.762
  circle A334 centre (-7.09, 32.79) radius 0.762
  circle A335 centre (-4.55, 30.25) radius 0.762
  circle A336 centre (-9.63, 30.25) radius 0.762
  circle A337 centre (-14.71, 30.25) radius 0.762
  circle A338 centre (-14.71, 25.17) radius 0.762
  circle A339 centre (-12.17, 22.63) radius 0.762
  circle A340 centre (-12.17, 27.71) radius 0.762
  circle A341 centre (-9.63, 25.17) radius 0.762
  circle A342 centre (-7.09, 22.63) radius 0.762
  circle A343 centre (-7.09, 27.71) radius 0.762
  circle A344 centre (-4.55, 25.17) radius 0.762
  circle A345 centre (-4.55, 20.09) radius 0.762
  circle A346 centre (-9.63, 20.09) radius 0.762
  circle A347 centre (-14.71, 20.09) radius 0.762
  circle A348 centre (-7.09, -33.25) radius 0.762
  circle A349 centre (-12.17, -33.25) radius 0.762
  circle A350 centre (-14.71, -30.71) radius 0.762
  circle A351 centre (-9.63, -30.71) radius 0.762
  circle A352 centre (-4.55, -30.71) radius 0.762
  circle A353 centre (-4.55, -25.63) radius 0.762
  circle A354 centre (-4.55, -20.55) radius 0.762
  circle A355 centre (-7.09, -23.09) radius 0.762
  circle A356 centre (-7.09, -28.17) radius 0.762
  circle A357 centre (-12.17, -28.17) radius 0.762
  circle A358 centre (-14.71, -25.63) radius 0.762
  circle A359 centre (-9.63, -25.63) radius 0.762
  circle A360 centre (-9.63, -20.55) radius 0.762
  circle A361 centre (-12.17, -23.09) radius 0.762
  circle A362 centre (-14.71, -20.55) radius 0.762
  circle A363 centre (-12.17, -18.01) radius 0.762
  circle A364 centre (-7.09, -18.01) radius 0.762
  circle A365 centre (-4.55, -15.47) radius 0.762
  circle A366 centre (-9.63, -15.47) radius 0.762
  circle A367 centre (-14.71, -15.47) radius 0.762
  circle A368 centre (-12.17, -12.93) radius 0.762
  circle A369 centre (-7.09, -12.93) radius 0.762
  circle A370 centre (-4.55, -10.39) radius 0.762
  circle A371 centre (-4.55, -5.31) radius 0.762
  circle A372 centre (-4.55, -0.23) radius 0.762
  circle A373 centre (-4.55, 4.85) radius 0.762
  circle A374 centre (-4.55, 9.93) radius 0.762
  circle A375 centre (-4.55, 15.01) radius 0.762
  circle A376 centre (-14.71, 17.55) radius 0.762
  circle A377 centre (-14.71, 12.47) radius 0.762
  circle A378 centre (-14.71, 7.39) radius 0.762
  circle A379 centre (-14.71, -0.23) radius 0.762
  circle A380 centre (-14.71, -2.77) radius 0.762
  circle A381 centre (-14.71, -7.85) radius 0.762
  circle A382 centre (-12.17, 17.55) radius 0.762
  circle A383 centre (-7.09, 17.55) radius 0.762
  circle A384 centre (-9.63, 15.01) radius 0.762
  circle A385 centre (-12.17, 12.47) radius 0.762
  circle A386 centre (-7.09, 12.47) radius 0.762
  circle A387 centre (-9.63, 9.93) radius 0.762
  circle A388 centre (-12.17, 7.39) radius 0.762
  circle A389 centre (-7.09, 7.39) radius 0.762
  circle A390 centre (-9.63, 4.85) radius 0.762
  circle A391 centre (-12.17, 2.31) radius 0.762
  circle A392 centre (-7.09, 2.31) radius 0.762
  circle A393 centre (-9.63, -10.39) radius 0.762
  circle A394 centre (-7.09, -7.85) radius 0.762
  circle A395 centre (-12.17, -7.85) radius 0.762
  circle A396 centre (-7.09, -2.77) radius 0.762
  circle A397 centre (-9.63, -0.23) radius 0.762
  circle A398 centre (-12.17, -2.77) radius 0.762
  circle A399 centre (-9.63, -5.31) radius 0.762
  line L5 (-2.35, 38.65) -> (-26.65, 38.65)
  line L6 (-26.65, 38.65) -> (-26.65, -41.65)
  line L7 (-26.65, -41.65) -> (-2.35, -41.65)
  line L8 (-2.35, -41.65) -> (-2.35, 38.65)
  point P0 (20.71, 0)
  point P1 (13.96, -1.27)
  dimension "d38" = 6.75
  constraint coincident L0.start origin
  constraint coincident L0 P0
  measures "d38" horizontal distance of P0 P1
sketch "Sketch7" plane through (0, 0, 9.7) normal (0, 0, 1) x (-1, 0, 0)
equation "d35 = ( 2.54 * 4 ) * 1 mm"
equation "d36 = ( -2.54 * 14 ) * 1 mm"
equation "d43 = ( 2.54 * 4 ) * 1 mm"
equation "d44 = ( -2.54 * 14 ) * 1 mm"
equation "d50 = ( -2.54 * 2 ) * 1 mm"
equation "d54 = ( 12 * 2.54 ) * 1 mm"
equation "d56 = ( 2.54 * 3 / 5 ) * 1 mm"
